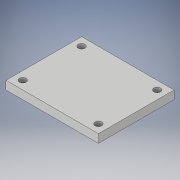
# Autodesk Inventor part: Spiegelhalter_klein
Saved by Autodesk Inventor 2018.3 (Build 223284000, 284)
## iProperties
Created: 2018-11-15
Part Number: Spiegelhalter_klein
Material: Generisch
Document SubType Name: Modeling
Designer: pgmadmin
Density: 1 g/cm^3
Appearance: Vorgabe
Author: pgmadmin
Autodesk Inventor part; units mm, degrees
ref_plane "YZ Plane" through (0, 0, 0) normal (1, 0, 0) x (0, 1, 0)
ref_plane "XZ Plane" through (0, 0, 0) normal (0, 1, 0) x (-1, 0, 0)
ref_plane "XY Plane" through (0, 0, 0) normal (0, 0, 1) x (1, 0, 0)
sketch "Skizze1" plane through (0, 0, 0) normal (0, 0, 1) x (1, 0, 0)
  line L0 (-27.5, -22.5) -> (27.5, -22.5)
  line L1 (27.5, -22.5) -> (27.5, 22.5)
  line L2 (27.5, 22.5) -> (-27.5, 22.5)
  line L3 (-27.5, 22.5) -> (-27.5, -22.5)
  line L4 (-27.5, -22.5) -> (27.5, 22.5) construction
  line L5 (27.5, -22.5) -> (-27.5, 22.5) construction
  point P0 (0, 0)
  point P1 (-22.5, 17.5)
  point P2 (22.5, 17.5)
  point P3 (22.5, -17.5)
  point P4 (-22.5, -17.5)
  dimension "d0" = 55
  dimension "d1" = 45
  dimension "d2" = 5
  dimension "d3" = 5
  dimension "d4" = 5
  dimension "d5" = 5
  dimension "d6" = 5
  dimension "d7" = 5
  dimension "d8" = 5
  dimension "d9" = 5
  constraints: 12 end point, 2 midpoint, 2 parallel, 1 horizontal, 1 perpendicular
  measures "d0" distance of L2.end L1.end
  measures "d1" distance between parallel lines of L0 L2
  measures "d2" distance from line of L2 point (-22.5, 17.5)
  measures "d3" distance from line of L3 point (-22.5, 17.5)
  measures "d4" distance from line of L2 point (22.5, 17.5)
  measures "d5" distance from line of L1 point (22.5, 17.5)
  measures "d6" distance from line of L1 point (22.5, -17.5)
  measures "d7" distance from line of L0 point (22.5, -17.5)
  measures "d8" distance from line of L0 point (-22.5, -17.5)
  measures "d9" distance from line of L3 point (-22.5, -17.5)
extrude "Extrusion1" add sketch "Skizze1" along normal blind 5
sketch "Skizze2" plane through (0, 0, 0) normal (0, 0, -1) x (-1, 0, 0)
  line L0 (27.5, 22.5) -> (27.5, -22.5) projected
  line L1 (-27.5, 22.5) -> (27.5, 22.5) projected
  line L2 (27.5, -22.5) -> (-27.5, -22.5) projected
  line L3 (-27.5, -22.5) -> (-27.5, 22.5) projected
  point P0 (0, 0)
  point P1 (22.5, 17.5)
  point P2 (22.5, -17.5)
  point P3 (-22.5, -17.5)
  point P4 (-22.5, 17.5)
  dimension "d12" = 5
  dimension "d13" = 5
  dimension "d14" = 5
  dimension "d15" = 5
  dimension "d16" = 5
  dimension "d17" = 5
  dimension "d18" = 5
  dimension "d19" = 5
  measures "d12" distance from line of L0 point (22.5, 17.5)
  measures "d13" distance from line of L1 point (22.5, 17.5)
  measures "d14" distance from line of point (22.5, -17.5) L0
  measures "d15" distance from line of L2 point (22.5, -17.5)
  measures "d16" distance from line of L2 point (-22.5, -17.5)
  measures "d17" distance from line of L3 point (-22.5, -17.5)
  measures "d18" distance from line of L1 point (-22.5, 17.5)
  measures "d19" distance from line of L3 point (-22.5, 17.5)
hole "Bohrung1" at (-22.5, 17.5, 0) at (-22.5, -17.5, 0) at (22.5, -17.5, 0) at (22.5, 17.5, 0) direction (0, 0, 1) diameter 4 end through all counterbore diameter 6.5 counterbore depth 2.25
